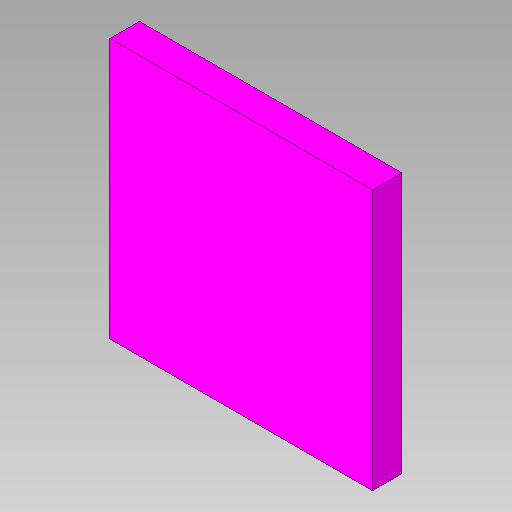
# Autodesk Inventor part: MSP430F5528IRGC
Saved by Autodesk Inventor 2020.1 (Build 241239000, 239)
## iProperties
Created: 2015-11-24
Part Number: MSP430F5528IRGC
Material: Generic
Document SubType Name: Modeling
Designer: PhillipD
Density: 1 g/cm^3
Appearance: RGC64, MSP430F5528IRGC
Author: PhillipD
Autodesk Inventor part; units mm, degrees
ref_plane "YZ Plane" through (0, 0, 0) normal (1, 0, 0) x (0, 1, 0)
ref_plane "XZ Plane" through (0, 0, 0) normal (0, 1, 0) x (-1, 0, 0)
ref_plane "XY Plane" through (0, 0, 0) normal (0, 0, 1) x (1, 0, 0)
sketch "RGC64, MSP430F5528IRGC_89" plane through (0, 0, 0) normal (0, 0, 1) x (1, 0, 0)
  line L0 (-4.4735, 4.4) -> (4.42, 4.4)
  line L1 (4.42, 4.4) -> (4.42, -4.42)
  line L2 (4.42, -4.42) -> (-4.4735, -4.42)
  line L3 (-4.4735, -4.42) -> (-4.4735, 4.4)
  constraints: 8 end point
extrude "Extrusion1" add sketch "RGC64, MSP430F5528IRGC_89" along normal blind 1
body "Solid1"
